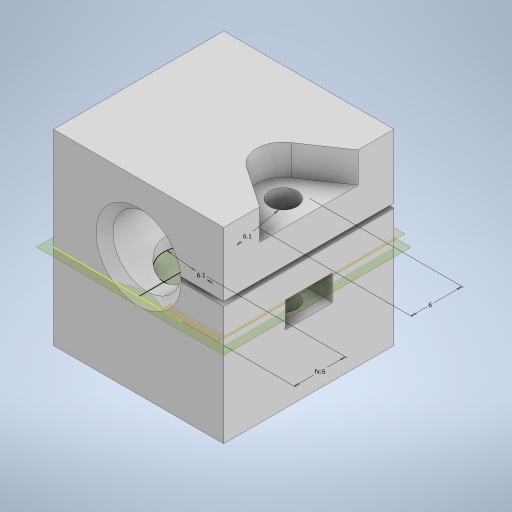
# Autodesk Inventor part: Y Rod Holder
Saved by Autodesk Inventor 2023.1 (Build 271208000, 208)
## iProperties
Created: 2022-10-29
Part Number: Y Rod Holder
Material: Generic
Document SubType Name: Modeling
Designer: nicol
Density: 1 g/cm^3
Appearance: Default
Author: nicol
Autodesk Inventor part; units mm, degrees
ref_plane "YZ Plane" through (0, 0, 0) normal (1, 0, 0) x (0, 1, 0)
ref_plane "XZ Plane" through (0, 0, 0) normal (0, 1, 0) x (-1, 0, 0)
ref_plane "XY Plane" through (0, 0, 0) normal (0, 0, 1) x (1, 0, 0)
sketch "Sketch1" plane through (0, 0, 0) normal (0, 0, 1) x (1, 0, 0)
  line L0 (0, 0) -> (20, 0)
  line L1 (20, 0) -> (20, 14)
  line L2 (20, 14) -> (0, 14)
  line L3 (0, 14) -> (0, 0)
  circle A0 centre (10, 14) radius 4
  line L4 (7.9329, 10) -> (16.1844, 10) construction
  line L5 (6, 14) -> (0, 14)
  line L6 (14, 14) -> (20, 14)
  line L7 (20, 14) -> (0, 14)
  line L8 (0, 14) -> (0, 22)
  line L9 (0, 22) -> (20, 22)
  line L10 (20, 22) -> (20, 14)
  line L11 (20, 13.5) -> (13.9686, 13.5)
  line L12 (13.9686, 13.5) -> (13.9686, 14.5)
  line L13 (13.9686, 14.5) -> (20, 14.5)
  line L14 (20, 14.5) -> (20, 13.5)
  point P0 (20, 7)
  point P1 (0, 7)
  point P2 (17, 14)
  point P3 (3, 14)
  point P4 (13.9686, 14)
  point P5 (0, 14)
  dimension "d0" = 8
  dimension "d1" = 10
  dimension "d2" = 20
  dimension "d5" = 8
  dimension "d6" = 1
  constraints: 30 end point, 6 midpoint, 6 parallel, 5 point on line, 4 horizontal, 3 perpendicular, 3 point on circle, 2 collinear, 1 centre point, 1 tangent
  measures "d0" diameter of A0
  measures "d1" distance between parallel lines of L0 L4
  measures "d2" distance of L1.end L2.end
  measures "d5" distance of L7.end L8.end
  measures "d6" distance between parallel lines of L13 L11
extrude "Extrusion1" add sketch "Sketch1" along normal blind 20 contours L3 L2 A0 L11 L1 L0 | L8 L9 L10 L13 A0 L2 | L11 A0 L2 L1
chamfer "Chamfer1" distance 1 angle 45 2 edges at (6.0079, 13.7495, 0) (6.0079, 13.7495, 20)
ref_plane "Work Plane1" through (20, 11, 20) normal (0, 1, 0) x (1, 0, 0)
sketch "Sketch2" plane through (0, 22, 0) normal (0, 1, 0) x (1, 0, 0)
  line L0 (15, -20) -> (14, -19) projected
  line L1 (20, -20) -> (15, -20) projected
  line L2 (20, 0) -> (20, -20) projected
  line L3 (20, 0) -> (15, 0) projected
  line L4 (14, -1) -> (15, 0) projected
  line L5 (14, -1) -> (14, -19) projected
  line L6 (14, -15.8523) -> (20, -15.8523)
  line L7 (15.4123, -7.25) -> (18.5877, -7.25)
  line L8 (18.5877, -7.25) -> (20.1754, -10) construction
  line L9 (20.1754, -10) -> (18.5877, -12.75) construction
  line L10 (18.5877, -12.75) -> (15.4123, -12.75)
  line L11 (15.4123, -12.75) -> (13.8246, -10)
  line L12 (13.8246, -10) -> (15.4123, -7.25)
  line L13 (18.5877, -12.75) -> (22.4339, -12.75)
  line L14 (22.4339, -12.75) -> (22.4339, -7.25)
  line L15 (22.4339, -7.25) -> (18.5877, -7.25)
  line L16 (18.5877, -7.25) -> (18.5877, -12.75) construction
  point P0 (0, 0)
  point P1 (17, -10)
  point P2 (20, -10)
  point P3 (17, -15.8523)
  point P4 (17, -10)
  dimension "d10" = 5.5
  constraints: 22 end point, 2 horizontal, 2 midpoint, 2 parallel, 2 perpendicular, 2 point on line, 1 coincident, 1 horizontal alignment, 1 vertical alignment, 13 other
  measures "d10" distance between parallel lines of L7 L10
extrude "Extrusion2" cut sketch "Sketch2" against normal blind 3 from surface at -11 contours L11 L12 L5 | L5 L12 L7 L15 L2 L13 L10 L11 | L2 L15 L14 L13
hole "Hole1" at (17, 22, 10) direction (0, -1, 0) diameter 3.2 end through all counterbore diameter 6.2 counterbore depth 3.58
chamfer "Chamfer2" distance 5 angle 45 2 edges at (20, 20.21, 9.219) (20, 20.21, 10.781)
ref_plane "Work Plane2" through (10, 10, 0) normal (0, -1, 0) x (1, 0, 0)
sketch "Sketch3" plane through (10, 10, 0) normal (0, -1, 0) x (1, 0, 0)
  line L0 (-5, 0) -> (5, 0) projected
  line L1 (5, 20) -> (-5, 20) projected
  line L2 (-10, 20) -> (10, 20) projected
  line L3 (0, 20) -> (0, 0)
  circle A0 centre (0, 14) radius 3.05
  circle A1 centre (0, 6) radius 3.05
  point P0 (-10, 0)
  point P1 (4.9749, 0)
  point P2 (4.9749, 20)
  dimension "d24" = 6.1
  dimension "d25" = 6.1
  dimension "d26" = 6
  dimension "d27" = 6
  constraints: 2 centre point, 2 coincident, 2 end point, 2 midpoint, 2 point on line
  measures "d24" diameter of A0
  measures "d25" diameter of A1
  measures "d26" distance of L3.end A1.centre
  measures "d27" distance from line of L1 A0.centre
extrude "Extrusion3" cut sketch "Sketch3" along normal blind 7 and the other way blind 2
hole "Hole2" at (10, 10, 6) at (10, 10, 14) direction (0, -1, 0) diameter 3.2 end through all
equation "\"d27\" = d26"
body "Solid1"
